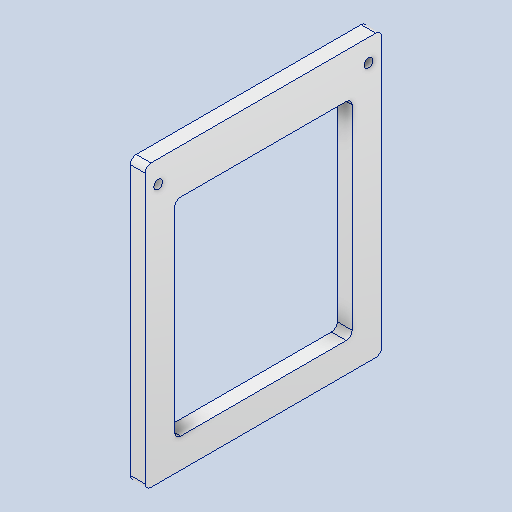
# Autodesk Inventor part: base_weel-v1-Plate-lider-C
Saved by Autodesk Inventor 2025.1 (Build 291241000, 241)
## iProperties
Created: 2024-10-25
Part Number: base_weel-v1-Plate-lider-C
Material: アルミニウム 6061
Document SubType Name: Modeling
Designer: haruy
Density: 2.7 g/cm^3
Appearance: アルミニウム - フラット
Author: haruy
Autodesk Inventor part; units mm, degrees
ref_plane "YZ Plane" through (0, 0, 0) normal (1, 0, 0) x (0, 1, 0)
ref_plane "XZ Plane" through (0, 0, 0) normal (0, 1, 0) x (-1, 0, 0)
ref_plane "XY Plane" through (0, 0, 0) normal (0, 0, 1) x (1, 0, 0)
sketch "スケッチ1" plane through (0, 0, 0) normal (1, 0, 0) x (0, 1, 0)
  line L0 (-151.1262, 435.4749) -> (478.8738, 435.4749)
  line L1 (478.8738, 435.4749) -> (478.8738, -194.5251)
  line L2 (478.8738, -194.5251) -> (-151.1262, -194.5251)
  line L3 (-151.1262, -194.5251) -> (-151.1262, 435.4749)
  line L4 (-151.1262, 435.4749) -> (478.8738, -194.5251) construction
  line L5 (478.8738, 435.4749) -> (-151.1262, -194.5251) construction
  line L6 (-151.1262, 342.6932) -> (-136.1262, 342.6932)
  line L7 (-136.1262, 342.6932) -> (-136.1262, -101.7433)
  line L8 (-136.1262, -101.7433) -> (-151.1262, -101.7433)
  line L9 (-151.1262, -101.7433) -> (-151.1262, 342.6932)
  line L10 (386.092, 435.4749) -> (-58.3445, 435.4749)
  line L11 (-58.3445, 435.4749) -> (-58.3445, 420.4749)
  line L12 (-58.3445, 420.4749) -> (386.092, 420.4749)
  line L13 (386.092, 420.4749) -> (386.092, 435.4749)
  line L14 (-58.3445, 420.4749) -> (-136.1262, 342.6932)
  line L15 (-136.1262, 342.6932) -> (-136.1262, 435.4749)
  line L16 (-58.3445, 420.4749) -> (-136.1262, 342.6932)
  line L17 (-136.1262, 342.6932) -> (-129.0552, 335.6221)
  line L18 (-129.0552, 335.6221) -> (-51.2734, 413.4039)
  line L19 (-51.2734, 413.4039) -> (-58.3445, 420.4749)
  line L20 (53.0814, 420.4749) -> (-136.1262, 231.2673)
  line L21 (53.0814, 420.4749) -> (-136.1262, 231.2673)
  line L22 (-136.1262, 231.2673) -> (-129.0552, 224.1962)
  line L23 (-129.0552, 224.1962) -> (60.1525, 413.4039)
  line L24 (60.1525, 413.4039) -> (53.0814, 420.4749)
  line L25 (163.8738, 120.4749) -> (-792.7235, 120.4749)
  line L26 (-58.3445, -179.5251) -> (-136.1262, -101.7433)
  line L27 (-136.1262, -101.7433) -> (-129.0552, -94.6723)
  line L28 (-129.0552, -94.6723) -> (-51.2734, -172.454)
  line L29 (-51.2734, -172.454) -> (-58.3445, -179.5251)
  line L30 (53.0814, -179.5251) -> (-136.1262, 9.6826)
  line L31 (-136.1262, 9.6826) -> (-129.0552, 16.7536)
  line L32 (-129.0552, 16.7536) -> (60.1525, -172.454)
  line L33 (60.1525, -172.454) -> (53.0814, -179.5251)
  circle A0 centre (163.8738, 120.4749) radius 400
  line L34 (-166.1262, 145.4749) -> (-216.1262, 145.4749)
  line L35 (-216.1262, 145.4749) -> (-216.1262, 95.4749)
  line L36 (-216.1262, 95.4749) -> (-166.1262, 95.4749)
  line L37 (-166.1262, 95.4749) -> (-166.1262, 145.4749)
  line L38 (163.8738, 120.4749) -> (163.8738, -510.4429)
  line L39 (386.092, 420.4749) -> (463.8738, 342.6932)
  line L40 (463.8738, 342.6932) -> (456.8027, 335.6221)
  line L41 (456.8027, 335.6221) -> (379.0209, 413.4039)
  line L42 (379.0209, 413.4039) -> (386.092, 420.4749)
  line L43 (274.6661, 420.4749) -> (463.8738, 231.2673)
  line L44 (463.8738, 231.2673) -> (456.8027, 224.1962)
  line L45 (456.8027, 224.1962) -> (267.5951, 413.4039)
  line L46 (267.5951, 413.4039) -> (274.6661, 420.4749)
  line L47 (456.8027, 16.7536) -> (267.5951, -172.454)
  line L48 (463.8738, 9.6826) -> (456.8027, 16.7536)
  line L49 (274.6661, -179.5251) -> (463.8738, 9.6826)
  line L50 (267.5951, -172.454) -> (274.6661, -179.5251)
  line L51 (463.8738, -101.7433) -> (456.8027, -94.6723)
  line L52 (386.092, -179.5251) -> (463.8738, -101.7433)
  line L53 (456.8027, -94.6723) -> (379.0209, -172.454)
  line L54 (379.0209, -172.454) -> (386.092, -179.5251)
  line L55 (-151.1262, 160.4749) -> (-231.1262, 160.4749)
  line L56 (-231.1262, 160.4749) -> (-231.1262, 150.4749)
  line L57 (-231.1262, 150.4749) -> (-151.1262, 150.4749)
  line L58 (-151.1262, 150.4749) -> (-151.1262, 160.4749)
  line L59 (-231.1262, 150.4749) -> (-221.1262, 150.4749)
  line L60 (-221.1262, 150.4749) -> (-221.1262, 120.4749)
  line L61 (-221.1262, 120.4749) -> (-231.1262, 120.4749)
  line L62 (-231.1262, 120.4749) -> (-231.1262, 150.4749)
  line L63 (463.8738, 342.6932) -> (478.8738, 342.6932)
  line L64 (478.8738, 342.6932) -> (478.8738, -101.7433)
  line L65 (478.8738, -101.7433) -> (463.8738, -101.7433)
  line L66 (463.8738, -101.7433) -> (463.8738, 342.6932)
  line L67 (-58.3445, -194.5251) -> (386.092, -194.5251)
  line L68 (386.092, -194.5251) -> (386.092, -179.5251)
  line L69 (386.092, -179.5251) -> (-58.3445, -179.5251)
  line L70 (-58.3445, -179.5251) -> (-58.3445, -194.5251)
  line L71 (378.3744, 409.2217) -> (452.6206, 334.9755)
  line L72 (452.6206, 334.9755) -> (417.8105, 300.1654)
  line L73 (417.8105, 300.1654) -> (343.5643, 374.4116)
  line L74 (343.5643, 374.4116) -> (378.3744, 409.2217)
  line L75 (478.8738, 435.4749) -> (163.8738, 120.4749)
  line L76 (478.8738, 265.4749) -> (-151.1262, 265.4749)
  line L77 (-151.1262, 265.4749) -> (-151.1262, 245.4749)
  line L78 (-151.1262, 245.4749) -> (478.8738, 245.4749)
  line L79 (478.8738, 245.4749) -> (478.8738, 265.4749)
  line L80 (478.8738, -24.5251) -> (-151.1262, -24.5251)
  line L81 (-151.1262, -4.5251) -> (478.8738, -4.5251)
  line L82 (478.8738, 265.4749) -> (498.8738, 265.4749)
  line L83 (498.8738, 265.4749) -> (498.8738, 285.4749)
  line L84 (498.8738, 285.4749) -> (478.8738, 285.4749)
  line L85 (478.8738, 285.4749) -> (478.8738, 265.4749)
  line L86 (478.8738, -24.5251) -> (498.8738, -24.5251)
  line L87 (498.8738, -24.5251) -> (498.8738, -44.5251)
  line L88 (498.8738, -44.5251) -> (478.8738, -44.5251)
  line L89 (478.8738, -44.5251) -> (478.8738, -24.5251)
  line L90 (498.8738, 285.4749) -> (511.3738, 285.4749)
  line L91 (504.3091, -44.5251) -> (494.3091, -44.5251)
  circle A1 centre (675.8738, 120.4749) radius 122.5
  line L92 (478.8738, 265.4749) -> (498.8738, 265.4749)
  line L93 (498.8738, 265.4749) -> (498.8738, 245.4749)
  line L94 (498.8738, 245.4749) -> (478.8738, 245.4749)
  line L95 (478.8738, 245.4749) -> (478.8738, 265.4749)
  line L96 (478.8738, -24.5251) -> (498.8738, -24.5251)
  line L97 (498.8738, -24.5251) -> (498.8738, -4.5251)
  line L98 (498.8738, -4.5251) -> (478.8738, -4.5251)
  line L99 (478.8738, -4.5251) -> (478.8738, -24.5251)
  line L100 (289.8738, 265.4749) -> (309.8738, 265.4749)
  line L101 (309.8738, 265.4749) -> (309.8738, 285.4749)
  line L102 (309.8738, 285.4749) -> (289.8738, 285.4749)
  line L103 (289.8738, 285.4749) -> (289.8738, 265.4749)
  line L104 (-129.0552, 335.6221) -> (-151.1262, 335.6221)
  circle A2 centre (-143.6262, 352.4749) radius 1.5
  circle A3 centre (-143.6262, 342.4749) radius 1.5
  line L105 (-136.1262, 362.4749) -> (-151.1262, 362.4749)
  line L106 (-58.3445, 427.9749) -> (-143.6262, 427.9749)
  line L107 (-143.6262, 427.9749) -> (-143.6262, 362.4749)
  circle A4 centre (-68.1262, 427.9749) radius 1.5
  circle A5 centre (-58.1262, 427.9749) radius 1.5
  line L108 (-78.1262, 435.4749) -> (-78.1262, 420.4749)
  line L109 (-58.3445, 420.4749) -> (-78.1262, 420.4749)
  circle A6 centre (-68.1262, -187.0251) radius 1.5
  circle A7 centre (-58.1262, -187.0251) radius 1.5
  circle A8 centre (-143.6262, -111.5251) radius 1.5
  circle A9 centre (-143.6262, -101.5251) radius 1.5
  line L110 (-136.1262, -121.5251) -> (-151.1262, -121.5251)
  line L111 (-78.1262, -194.5251) -> (-78.1262, -179.5251)
  line L112 (405.8738, 435.4749) -> (405.8738, 420.4749)
  circle A10 centre (395.8738, 427.9749) radius 1.5
  circle A11 centre (385.8738, 427.9749) radius 1.5
  line L113 (463.8738, 362.4749) -> (478.8738, 362.4749)
  circle A12 centre (471.3738, 352.4749) radius 1.5
  circle A13 centre (471.3738, 342.4749) radius 1.5
  line L114 (463.8738, -121.5251) -> (478.8738, -121.5251)
  circle A14 centre (471.3738, -111.5251) radius 1.5
  circle A15 centre (471.3738, -101.5251) radius 1.5
  line L115 (405.8738, -194.5251) -> (405.8738, -179.5251)
  circle A16 centre (395.8738, -187.0251) radius 1.5
  circle A17 centre (385.8738, -187.0251) radius 1.5
  line L116 (-136.1262, -101.7433) -> (-136.1262, -121.5251)
  line L117 (-58.3445, -179.5251) -> (-78.1262, -179.5251)
  line L118 (405.8738, -179.5251) -> (386.092, -179.5251)
  line L119 (463.8738, -101.7433) -> (463.8738, -121.5251)
  line L120 (463.8738, 362.4749) -> (463.8738, 342.6932)
  line L121 (386.092, 420.4749) -> (405.8738, 420.4749)
  circle A18 centre (-129.0552, 342.6932) radius 1.5
  circle A19 centre (-121.9841, 349.7643) radius 1.5
  circle A20 centre (-129.0552, 231.2673) radius 1.5
  circle A21 centre (-121.9841, 238.3384) radius 1.5
  circle A22 centre (-65.4156, 406.3328) radius 1.5
  circle A23 centre (-58.3445, 413.4039) radius 1.5
  circle A24 centre (46.0103, 406.3328) radius 1.5
  circle A25 centre (53.0814, 413.4039) radius 1.5
  circle A26 centre (-58.3445, -172.454) radius 1.5
  circle A27 centre (-65.4156, -165.3829) radius 1.5
  circle A28 centre (53.0814, -172.454) radius 1.5
  circle A29 centre (46.0103, -165.3829) radius 1.5
  circle A30 centre (-129.0552, -101.7433) radius 1.5
  circle A31 centre (-121.9841, -108.8144) radius 1.5
  circle A32 centre (-121.9841, 2.6115) radius 1.5
  circle A33 centre (-129.0552, 9.6826) radius 1.5
  circle A34 centre (456.8027, 9.6826) radius 1.5
  circle A35 centre (449.7316, 2.6115) radius 1.5
  circle A36 centre (456.8027, -101.7433) radius 1.5
  circle A37 centre (449.7316, -108.8144) radius 1.5
  circle A38 centre (393.1631, -165.3829) radius 1.5
  circle A39 centre (386.092, -172.454) radius 1.5
  circle A40 centre (281.7372, -165.3829) radius 1.5
  circle A41 centre (274.6661, -172.454) radius 1.5
  circle A42 centre (449.7316, 238.3384) radius 1.5
  circle A43 centre (456.8027, 231.2673) radius 1.5
  circle A44 centre (456.8027, 342.6932) radius 1.5
  circle A45 centre (449.7316, 349.7643) radius 1.5
  circle A46 centre (393.1631, 406.3328) radius 1.5
  circle A47 centre (386.092, 413.4039) radius 1.5
  circle A48 centre (274.6661, 413.4039) radius 1.5
  circle A49 centre (281.7372, 406.3328) radius 1.5
  circle A50 centre (-143.6262, 231.049) radius 1.5
  circle A51 centre (-143.6262, 241.049) radius 1.5
  circle A52 centre (43.2996, 427.9749) radius 1.5
  circle A53 centre (53.2996, 427.9749) radius 1.5
  circle A54 centre (-143.6262, 9.9008) radius 1.5
  circle A55 centre (-143.6262, -0.0992) radius 1.5
  circle A56 centre (43.2996, -187.0251) radius 1.5
  circle A57 centre (53.2996, -187.0251) radius 1.5
  circle A58 centre (274.4479, 427.9749) radius 1.5
  circle A59 centre (284.4479, 427.9749) radius 1.5
  circle A60 centre (471.3738, 241.049) radius 1.5
  circle A61 centre (471.3738, 231.049) radius 1.5
  circle A62 centre (471.3738, -0.0992) radius 1.5
  circle A63 centre (471.3738, 9.9008) radius 1.5
  circle A64 centre (284.4479, -187.0251) radius 1.5
  circle A65 centre (274.4479, -187.0251) radius 1.5
  circle A66 centre (471.3738, 255.4749) radius 1.5
  circle A67 centre (471.3738, -14.5251) radius 1.5
  circle A68 centre (-143.6262, -14.5251) radius 1.5
  circle A69 centre (-143.6262, 255.4749) radius 1.5
  circle A70 centre (314.8738, 255.4749) radius 1.5
  circle A71 centre (314.8738, -14.5251) radius 1.5
  circle A72 centre (-211.1262, 140.4749) radius 1.5
  line L122 (-191.1262, 145.4749) -> (-191.1262, 95.4749)
  circle A73 centre (-211.1262, 100.4749) radius 1.5
  circle A74 centre (-171.1262, 140.4749) radius 1.5
  circle A75 centre (-171.1262, 100.4749) radius 1.5
  circle A76 centre (-143.6262, 120.4749) radius 1.5
  circle A77 centre (-143.6262, 156.049) radius 1.5
  circle A78 centre (-171.1262, 155.4749) radius 1.5
  circle A79 centre (-211.1262, 155.4749) radius 1.5
  circle A80 centre (-226.1262, 135.4749) radius 1.5
  circle A81 centre (-226.1262, 105.4749) radius 1.5
  line L123 (-231.1262, 120.4749) -> (-231.1262, 90.4749)
  line L124 (-231.1262, 90.4749) -> (-151.1262, 90.4749)
  line L125 (-221.1262, 90.4749) -> (-221.1262, 120.4749)
  line L126 (-151.1262, 80.4749) -> (-231.1262, 80.4749)
  line L127 (-231.1262, 80.4749) -> (-231.1262, 90.4749)
  circle A82 centre (-211.1262, 85.4749) radius 1.5
  circle A83 centre (-171.1262, 85.4749) radius 1.5
  circle A84 centre (-143.6262, 84.9008) radius 1.5
  circle A85 centre (-191.1262, 120.4749) radius 10
  line L128 (-216.1262, 145.4749) -> (-191.1262, 120.4749)
  line L129 (-219.6618, 141.9394) -> (-194.6618, 116.9394)
  line L130 (-219.6618, 141.9394) -> (-221.1262, 143.4039)
  line L131 (-212.5907, 149.0105) -> (-187.5907, 124.0105)
  line L132 (-212.5907, 149.0105) -> (-214.0552, 150.4749)
  line L133 (-212.5907, 91.9394) -> (-187.5907, 116.9394)
  line L134 (-219.6618, 99.0105) -> (-194.6618, 124.0105)
  line L135 (-169.6618, 149.0105) -> (-194.6618, 124.0105)
  line L136 (-169.6618, 91.9394) -> (-194.6618, 116.9394)
  line L137 (-219.6618, 99.0105) -> (-221.1262, 97.546)
  line L138 (-212.5907, 91.9394) -> (-214.0552, 90.4749)
  line L139 (-169.6618, 149.0105) -> (-168.1973, 150.4749)
  line L140 (-169.6618, 91.9394) -> (-168.1973, 90.4749)
  line L141 (-151.1262, 160.4749) -> (-136.1262, 160.4749)
  line L142 (-151.1262, 80.4749) -> (-136.1262, 80.4749)
  line L143 (-151.1262, 150.4749) -> (-136.1262, 150.4749)
  line L144 (-151.1262, 90.4749) -> (-136.1262, 90.4749)
  point P0 (0, 0)
  point P1 (-151.1262, -24.5251)
  point P2 (478.8738, -4.5251)
  point P3 (-151.1262, 265.4749)
  dimension "d0" = 3
  dimension "d1" = 68
  dimension "d2" = 7.5
  dimension "d3" = 3
  dimension "d4" = 10
  dimension "d5" = 7.5
  dimension "d6" = 10
  dimension "d7" = 3
  dimension "d8" = 3
  dimension "d9" = 10
  dimension "d10" = 68
  dimension "d11" = 7.5
  dimension "d12" = 7.5
  dimension "d13" = 10
  dimension "d14" = 3
  dimension "d15" = 3
  dimension "d16" = 5
  dimension "d17" = 10
  dimension "d18" = 5
  dimension "d19" = 5
  dimension "d20" = 3
  dimension "d21" = 3
  dimension "d22" = 5
  dimension "d23" = 10
  dimension "d24" = 5
  dimension "d25" = 5
  dimension "d26" = 0.2182
  dimension "d27" = 3
  dimension "d28" = 7.5
  dimension "d29" = 0.2182
  dimension "d30" = 3
  dimension "d31" = 10
  dimension "d32" = 7.5
  dimension "d33" = 3
  dimension "d34" = 7.5
  dimension "d35" = 10
  dimension "d36" = 3
  dimension "d37" = 5
  dimension "d38" = 10
  dimension "d39" = 3
  dimension "d40" = 5
  dimension "d41" = 5
  dimension "d42" = 3
  dimension "d43" = 3
  dimension "d44" = 7.5
  dimension "d45" = 7.5
  dimension "d46" = 75
  dimension "d47" = 3
  dimension "d48" = 3
  dimension "d49" = 5
  dimension "d50" = 5
  dimension "d51" = 20
  dimension "d52" = 20
  dimension "d53" = 3
  dimension "d54" = 15
  dimension "d55" = 5
  dimension "d56" = 20
  dimension "d57" = 5
  dimension "d58" = 5
  constraints: 290 end point, 92 symmetric about line, 86 centre point, 11 point on line, 7 perpendicular, 6 midpoint, 4 collinear, 3 horizontal, 3 parallel, 2 vertical, 65 other
  measures "d0" diameter of A2
  measures "d1" distance from line of A2.centre L12
  measures "d2" distance from line of A2.centre L3
  measures "d3" diameter of A3
  measures "d4" distance of A2.centre A3.centre
  measures "d5" distance from line of A3.centre L3
  measures "d6" distance from line of L105 A2.centre
  measures "d7" diameter of A4
  measures "d8" diameter of A5
  measures "d9" distance of A4.centre A5.centre
  measures "d10" horizontal distance of L105.start A4.centre
  measures "d11" distance from line of A4.centre L0
  measures "d12" distance from line of L10 A5.centre
  measures "d13" distance from line of L108 A4.centre
  measures "d14" diameter of A18
  measures "d15" diameter of A19
  measures "d16" distance from line of A18.centre L17
  measures "d17" distance of A19.centre A18.centre
  measures "d18" distance from line of A18.centre L14
  measures "d19" distance from line of A19.centre L14
  measures "d20" diameter of A20
  measures "d21" diameter of A21
  measures "d22" distance from line of A20.centre L22
  measures "d23" distance of A21.centre A20.centre
  measures "d24" distance from line of A20.centre L20
  measures "d25" distance from line of A21.centre L20
  measures "d26" vertical distance of A3.centre A18.centre
  measures "d27" diameter of A50
  measures "d28" distance from line of A50.centre L3
  measures "d29" vertical distance of A50.centre A20.centre
  measures "d30" diameter of A51
  measures "d31" distance of A50.centre A51.centre
  measures "d32" distance from line of L3 A51.centre
  measures "d33" diameter of A66
  measures "d34" distance from line of A66.centre L1
  measures "d35" distance from line of A66.centre L76
  measures "d36" diameter of A70
  measures "d37" distance from line of A70.centre L101
  measures "d38" distance from line of L76 A70.centre
  measures "d39" diameter of A72
  measures "d40" distance from line of A72.centre L35
  measures "d41" distance from line of A72.centre L34
  measures "d42" diameter of A76
  measures "d43" diameter of A77
  measures "d44" distance from line of A76.centre L9
  measures "d45" distance from line of A77.centre L9
  measures "d46" distance of A77.centre A50.centre
  measures "d47" diameter of A78
  measures "d48" diameter of A79
  measures "d49" distance from line of L55 A78.centre
  measures "d50" distance from line of A79.centre L55
  measures "d51" distance from line of A79.centre L56
  measures "d52" distance from line of A78.centre L9
  measures "d53" diameter of A80
  measures "d54" distance from line of A80.centre L59
  measures "d55" distance from line of A80.centre L62
  measures "d56" diameter of A85
  measures "d57" distance between parallel lines of L128 L129
  measures "d58" distance between parallel lines of L128 L131
extrude "押し出し1" add sketch "スケッチ1" against normal blind 5 contours L62 L57 L60 L25 | L25 L125 L124 L123 | L56 L55 L3 L57 | L124 L3 L126 L127 | L141 L7 L143 L3 | L3 L144 L7 L142 | L143 L7 L25 A76 L3 | L3 L25 A76 L7 L144 | A76 L25 | L25 A76 | A78 | A79 | A80 | A81 | A82 | A83
fillet "フィレット1" radius 2 8 edges at (-2.5, -231.1262, 160.4749) (-2.5, -231.1262, 80.4749) (-2.5, -136.1262, 80.4749) (-2.5, -136.1262, 160.4749) (-2.5, -221.1262, 90.4749) (-2.5, -221.1262, 150.4749) (-2.5, -151.1262, 90.4749) (-2.5, -151.1262, 150.4749)
equation "\"d5\" = d2"
equation "\"d12\" = d11"
equation "\"d19\" = d18"
equation "\"d25\" = d24"
equation "\"d29\" = d26"
equation "\"d32\" = d28"
equation "\"d45\" = d44"
equation "\"d50\" = d49"
